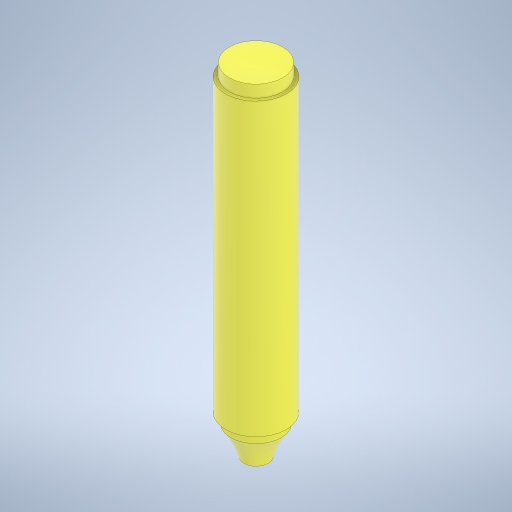
# Autodesk Inventor part: Marcador
Saved by Autodesk Inventor 2023.1 (Build 271208000, 208)
## iProperties
Created: 2022-08-24
Part Number: Marcador
Material: PC/ABS Plastic
Document SubType Name: Modeling
Designer: Daniel Peña
Density: 0.357273 g/cm^3
Appearance: Smooth - Yellow
Author: Daniel Peña
Autodesk Inventor part; units mm, degrees
ref_plane "YZ Plane" through (0, 0, 0) normal (1, 0, 0) x (0, 1, 0)
ref_plane "XZ Plane" through (0, 0, 0) normal (0, 1, 0) x (-1, 0, 0)
ref_plane "XY Plane" through (0, 0, 0) normal (0, 0, 1) x (1, 0, 0)
sketch "Sketch1" plane through (0, 0, 0) normal (0, 0, 1) x (1, 0, 0)
  line L0 (8.36, 75.283) -> (9.5, 75.283)
  line L1 (9.5, 75.283) -> (9.5, -15.717)
  line L2 (0, -27.717) -> (0, 80.883)
  line L3 (9.5, -15.717) -> (7.9, -15.717)
  line L4 (7.9, -15.717) -> (7.9, -18.717)
  arc A0 (7.9, -18.717) -> (3.825, -27.717) centre (31.6668, -34.9007) ccw
  line L5 (3.825, -27.717) -> (0, -27.717)
  line L6 (8.36, 75.283) -> (8.36, 79.083)
  line L7 (8.36, 79.083) -> (7.9, 79.083)
  arc A1 (8.36, 79.083) -> (0, 80.883) centre (0.6677, 63.6703) ccw
  point P0 (0, 0)
  dimension "d0" = 19
  dimension "d1" = 91
  dimension "d2" = 15.8
  dimension "d3" = 3
  dimension "d6" = 7.65
  dimension "d7" = 9
  dimension "d8" = 3.8
  constraints: 16 end point, 4 horizontal, 4 point on circle, 2 centre point, 2 perpendicular, 1 parallel, 1 point on line, 1 vertical
  measures "d0" diameter of L1 L2
  measures "d1" distance of L0.end L1.end
  measures "d2" diameter of L4 L2
  measures "d3" distance of L3.end L4.end
  measures "d6" diameter of L5.start L2
  measures "d7" vertical distance of L4.end L5.start
  measures "d8" distance of L0.start L6.end
revolve "Revolution1" add sketch "Sketch1" angle 360 about axis through (0, -27.717, 0) along (0, 1, 0)
body "Solid1"
